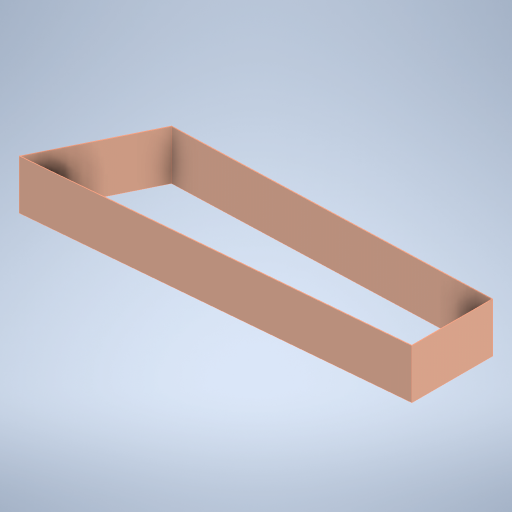
# Autodesk Inventor part: Fence
Saved by Autodesk Inventor 2024 (Build 280153020, 153B)
## iProperties
Created: 2023-06-05
Part Number: Fence
Material: Wood (Southern Pine)
Document SubType Name: Modeling
Designer: Tom
Density: 0.420735 g/cm^3
Appearance: Southern Pine
Author: Tom
Autodesk Inventor part; units mm, degrees
ref_plane "YZ Plane" through (0, 0, 0) normal (1, 0, 0) x (0, 1, 0)
ref_plane "XZ Plane" through (0, 0, 0) normal (0, 1, 0) x (-1, 0, 0)
ref_plane "XY Plane" through (0, 0, 0) normal (0, 0, 1) x (1, 0, 0)
sketch "Sketch1" plane through (0, 0, 0) normal (0, 1, 0) x (-1, 0, 0)
  line L0 (0, 0) -> (62323.0931, 5540.2604)
  line L1 (62323.0931, 5540.2604) -> (53646.5331, -12152.9626)
  line L2 (0, 0) -> (0, -14007.592)
  line L3 (0, -14007.592) -> (53646.5331, -12152.9626)
  line L4 (53578.1109, -12047.3135) -> (62141.8128, 5415.7697)
  line L5 (62141.8128, 5415.7697) -> (107.95, -98.7794)
  line L6 (107.95, -98.7794) -> (107.95, -13895.8455)
  line L7 (107.95, -13895.8455) -> (53578.1109, -12047.3135)
  dimension "d0" = 62568.8614
  dimension "d3" = 53678.582
  dimension "d5" = 95.08
  dimension "d6" = 88.02
  dimension "d7" = 14007.592
  dimension "d8" = 107.95
  constraints: 16 end point, 1 vertical, 3 other
  measures "d0" distance of L0.start L0.end
  measures "d3" distance of L2.end L1.end
  measures "d5" angle of L2 L0
  measures "d6" angle of L2 L3
  measures "d7" distance of L0.start L2.end
  measures "d8" distance between parallel lines of L1 L4
extrude "Extrusion1" add sketch "Sketch1" along normal blind 8534.4
body "Solid1"
